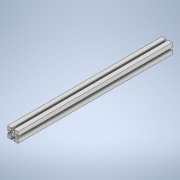
# Autodesk Inventor part: Axel_arch3
Saved by Autodesk Inventor 2020 (Build 240168000, 168)
## iProperties
Created: 2022-06-13
Part Number: Axel_arch3
Material: 일반
Document SubType Name: Modeling
Designer: samsung
Density: 1 g/cm^3
Appearance: 기본값
Author: samsung
Autodesk Inventor part; units mm, degrees
ref_plane "YZ Plane" through (0, 0, 0) normal (1, 0, 0) x (0, 1, 0)
ref_plane "XZ Plane" through (0, 0, 0) normal (0, 1, 0) x (-1, 0, 0)
ref_plane "작업 평면3" through (0, 0, 0) normal (0, 0, 1) x (1, 0, 0)
sketch "스케치4" plane through (0, 0, 0) normal (0, 0, 1) x (1, 0, 0)
  line L0 (-20, 182) -> (10, 182)
  line L1 (10, 182) -> (-20, 182)
  line L2 (-20, 182) -> (-20, 152)
  line L3 (-20, 152) -> (10, 152)
  line L4 (10, 152) -> (10, 182)
  line L5 (-20, 152) -> (-10, 152)
  line L6 (-10, 152) -> (-10, 162)
  line L7 (-10, 162) -> (-20, 162)
  line L8 (-20, 162) -> (-20, 152)
  line L9 (-20, 182) -> (-10, 182)
  line L10 (-10, 182) -> (-10, 172)
  line L11 (-10, 172) -> (-20, 172)
  line L12 (-20, 172) -> (-20, 182)
  line L13 (10, 152) -> (0, 152)
  line L14 (0, 152) -> (0, 162)
  line L15 (0, 162) -> (10, 162)
  line L16 (10, 162) -> (10, 152)
  line L17 (10, 182) -> (0, 182)
  line L18 (0, 182) -> (0, 172)
  line L19 (0, 172) -> (10, 172)
  line L20 (10, 172) -> (10, 182)
  line L21 (-18, 160) -> (-12, 160)
  line L22 (-12, 160) -> (-12, 154)
  line L23 (-12, 154) -> (-18, 154)
  line L24 (-18, 154) -> (-18, 160)
  line L25 (-18, 174) -> (-12, 174)
  line L26 (-12, 174) -> (-12, 180)
  line L27 (-12, 180) -> (-18, 180)
  line L28 (-18, 180) -> (-18, 174)
  line L29 (2, 160) -> (2, 154)
  line L30 (2, 154) -> (8, 154)
  line L31 (8, 154) -> (8, 160)
  line L32 (8, 160) -> (2, 160)
  line L33 (2, 174) -> (2, 180)
  line L34 (2, 180) -> (8, 180)
  line L35 (8, 180) -> (8, 174)
  line L36 (8, 174) -> (2, 174)
  line L37 (-10, 152) -> (-8, 152)
  line L38 (-8, 152) -> (-8, 154)
  line L39 (-8, 154) -> (-10, 154)
  line L40 (-10, 154) -> (-10, 152)
  line L41 (0, 152) -> (-2, 152)
  line L42 (-2, 152) -> (-2, 154)
  line L43 (-2, 154) -> (0, 154)
  line L44 (0, 154) -> (0, 152)
  line L45 (0, 182) -> (-2, 182)
  line L46 (-2, 182) -> (-2, 180)
  line L47 (-2, 180) -> (0, 180)
  line L48 (0, 180) -> (0, 182)
  line L49 (-10, 182) -> (-8, 182)
  line L50 (-8, 182) -> (-8, 180)
  line L51 (-8, 180) -> (-10, 180)
  line L52 (-10, 180) -> (-10, 182)
  line L53 (10, 162) -> (8, 162)
  line L54 (8, 162) -> (8, 164)
  line L55 (8, 164) -> (10, 164)
  line L56 (10, 164) -> (10, 162)
  line L57 (10, 172) -> (8, 172)
  line L58 (8, 172) -> (8, 170)
  line L59 (8, 170) -> (10, 170)
  line L60 (10, 170) -> (10, 172)
  line L61 (-20, 162) -> (-18, 162)
  line L62 (-18, 162) -> (-18, 164)
  line L63 (-18, 164) -> (-20, 164)
  line L64 (-20, 164) -> (-20, 162)
  line L65 (-20, 172) -> (-18, 172)
  line L66 (-18, 172) -> (-18, 170)
  line L67 (-18, 170) -> (-20, 170)
  line L68 (-20, 170) -> (-20, 172)
  line L69 (0, 162) -> (-10, 162)
  line L70 (-10, 162) -> (-10, 172)
  line L71 (-10, 172) -> (0, 172)
  line L72 (0, 172) -> (0, 162)
  line L73 (0, 162) -> (-10, 172) construction
  line L74 (-10, 162) -> (0, 172) construction
  line L75 (-8.5858, 162) -> (-10, 163.4142)
  line L76 (-10, 163.4142) -> (-11.4142, 162)
  line L77 (-11.4142, 162) -> (-10, 160.5858)
  line L78 (-10, 160.5858) -> (-8.5858, 162)
  line L79 (-8.5858, 162) -> (-11.4142, 162) construction
  line L80 (-10, 163.4142) -> (-10, 160.5858) construction
  line L81 (-8.5858, 172) -> (-10, 173.4142)
  line L82 (-10, 173.4142) -> (-11.4142, 172)
  line L83 (-11.4142, 172) -> (-10, 170.5858)
  line L84 (-10, 170.5858) -> (-8.5858, 172)
  line L85 (-8.5858, 172) -> (-11.4142, 172) construction
  line L86 (-10, 173.4142) -> (-10, 170.5858) construction
  line L87 (0, 170.5858) -> (1.4142, 172)
  line L88 (1.4142, 172) -> (0, 173.4142)
  line L89 (0, 173.4142) -> (-1.4142, 172)
  line L90 (-1.4142, 172) -> (0, 170.5858)
  line L91 (0, 170.5858) -> (0, 173.4142) construction
  line L92 (1.4142, 172) -> (-1.4142, 172) construction
  line L93 (0, 163.4142) -> (1.4142, 162)
  line L94 (1.4142, 162) -> (0, 160.5858)
  line L95 (0, 160.5858) -> (-1.4142, 162)
  line L96 (-1.4142, 162) -> (0, 163.4142)
  line L97 (0, 163.4142) -> (0, 160.5858) construction
  line L98 (1.4142, 162) -> (-1.4142, 162) construction
  line L99 (-2, 170) -> (-8, 170)
  line L100 (-8, 170) -> (-8, 164)
  line L101 (-8, 164) -> (-2, 164)
  line L102 (-2, 164) -> (-2, 170)
  point P0 (-5, 167)
  point P1 (0, 160.5858)
  point P2 (0, 173.4142)
  dimension "d19" = 30
  dimension "d20" = 10
  dimension "d21" = 10
  dimension "d22" = 10
  dimension "d23" = 10
  dimension "d24" = 10
  dimension "d25" = 10
  dimension "d26" = 10
  dimension "d27" = 10
  dimension "d28" = 2
  dimension "d29" = 2
  dimension "d30" = 2
  dimension "d31" = 2
  dimension "d32" = 2
  dimension "d33" = 2
  dimension "d34" = 2
  dimension "d35" = 2
  dimension "d36" = 2
  dimension "d37" = 2
  dimension "d38" = 2
  dimension "d39" = 2
  dimension "d40" = 2
  dimension "d41" = 2
  dimension "d42" = 2
  dimension "d43" = 2
  dimension "d44" = 2
  dimension "d45" = 2
  dimension "d46" = 2
  dimension "d47" = 2
  dimension "d98" = 2
  dimension "d99" = 2
  dimension "d100" = 2
  dimension "d101" = 2
  dimension "d102" = 2
  dimension "d103" = 2
  dimension "d104" = 2
  dimension "d105" = 2
  dimension "d116" = 2
  constraints: 206 end point, 48 parallel, 23 perpendicular, 15 horizontal, 10 midpoint, 15 other
  measures "d19" distance of L2.end L1.end
  measures "d20" distance of L7.end L6.end
  measures "d21" distance of L6.end L5.end
  measures "d22" distance of L10.end L11.end
  measures "d23" distance of L9.end L10.end
  measures "d24" distance of L14.end L15.end
  measures "d25" distance of L13.end L14.end
  measures "d26" distance of L19.end L18.end
  measures "d27" distance of L18.end L17.end
  measures "d28" distance between parallel lines of L7 L21
  measures "d29" distance between parallel lines of L11 L25
  measures "d30" distance between parallel lines of L14 L29
  measures "d31" distance between parallel lines of L18 L33
  measures "d32" distance of L39.end L38.end
  measures "d33" distance of L38.end L37.end
  measures "d34" distance of L42.end L43.end
  measures "d35" distance of L41.end L42.end
  measures "d36" distance of L47.end L46.end
  measures "d37" distance of L46.end L45.end
  measures "d38" distance of L50.end L51.end
  measures "d39" distance of L49.end L50.end
  measures "d40" distance of L54.end L55.end
  measures "d41" distance of L53.end L54.end
  measures "d42" distance of L59.end L58.end
  measures "d43" distance of L58.end L57.end
  measures "d44" distance of L63.end L62.end
  measures "d45" distance of L62.end L61.end
  measures "d46" distance of L66.end L67.end
  measures "d47" distance of L65.end L66.end
  measures "d98" distance of L75.start L75.end
  measures "d99" distance of L76.end L75.end
  measures "d100" distance of L81.start L81.end
  measures "d101" distance of L82.end L81.end
  measures "d102" distance of L87.start L87.end
  measures "d103" distance of L88.end L87.end
  measures "d104" distance of L93.start L93.end
  measures "d105" distance of L93.end L94.end
  measures "d116" distance between parallel lines of L71 L99
extrude "돌출7" add sketch "스케치4" against normal blind 127 contours L0 L10 L82 L11 L2 | L0 L50 L51 L10 | L11 L66 L67 L2 | L0 L18 L47 L46 | L81 L71 L10 | L10 L11 L82 | L63 L62 L7 L2 | L11 L70 L83 | L0 L4 L19 L88 L18 | L71 L84 L70 | L71 L90 L72 L96 L69 L75 L70 L84 | L7 L77 L6 L3 L2 | L89 L18 L71 | L71 L72 L90 | L75 L69 L70 | L70 L7 L76 | L4 L59 L58 L19 | L88 L19 L18 | L19 L87 L72 | L6 L39 L38 L3 | L7 L6 L77 | L69 L78 L6 | L93 L15 L72 | L72 L69 L96 | L69 L14 L95 | L4 L15 L54 L55 | L15 L94 L14 | L15 L4 L3 L14 L94 | L42 L43 L14 L3
sketch "스케치11" plane through (-20, 152, 0) normal (0, -1, 0) x (1, 0, 0)
  line L0 (18, 0) -> (30, 0) projected
  line L1 (18, 0) -> (18, -127) projected
  line L2 (30, -127) -> (18, -127) projected
  line L3 (30, 0) -> (30, -127) projected
  line L4 (0, 0) -> (12, 0) projected
  line L5 (0, 0) -> (0, -127) projected
  line L6 (12, -127) -> (0, -127) projected
  line L7 (12, 0) -> (12, -127) projected
  line L8 (0, 0) -> (12, 0) projected
  line L9 (30, 0) -> (30, -127) projected
  line L10 (0, 0) -> (30, 0)
  line L11 (30, 0) -> (30, -25)
  line L12 (30, -25) -> (0, -25)
  line L13 (0, -25) -> (0, 0)
  line L14 (30, -127) -> (0, -127)
  line L15 (0, -127) -> (0, -102)
  line L16 (0, -102) -> (30, -102)
  line L17 (30, -102) -> (30, -127)
  point P0 (20, 0)
  point P1 (15, -6.5)
  point P2 (15, -18.5)
  point P3 (15, -108.5)
  point P4 (15, -120.5)
  dimension "d117" = 25
  dimension "d118" = 25
  dimension "d119" = 6.5
  dimension "d120" = 6.5
  dimension "d121" = 6.5
  dimension "d122" = 6.5
  constraints: 16 end point, 4 parallel, 2 horizontal, 2 perpendicular, 2 point on line
  measures "d117" distance of L10.end L11.end
  measures "d118" distance of L14.end L15.end
  measures "d119" distance from line of point (15, -6.5) L10
  measures "d120" distance from line of L12 point (15, -18.5)
  measures "d121" distance from line of L16 point (15, -108.5)
  measures "d122" distance from line of L14 point (15, -120.5)
hole "구멍1" at (-5, 152, -6.5) at (-5, 152, -18.5) at (-5, 152, -108.5) at (-5, 152, -120.5) direction (0, 1, 0) diameter 6 end through all
sketch "스케치12" plane through (0, 0, 0) normal (0, 0, 1) x (1, 0, 0)
  line L0 (-1.4142, 162) -> (0, 160.5858) projected
  line L1 (0, 160.5858) -> (0, 154) projected
  line L2 (0, 154) -> (-2, 154) projected
  line L3 (-2, 154) -> (-2, 152) projected
  line L4 (-2, 152) -> (10, 152) projected
  line L5 (10, 152) -> (10, 164) projected
  line L6 (10, 164) -> (8, 164) projected
  line L7 (8, 164) -> (8, 162) projected
  line L8 (8, 162) -> (1.4142, 162) projected
  line L9 (1.4142, 162) -> (0, 163.4142) projected
  line L10 (0, 163.4142) -> (0, 170.5858) projected
  line L11 (0, 170.5858) -> (1.4142, 172) projected
  line L12 (1.4142, 172) -> (8, 172) projected
  line L13 (8, 172) -> (8, 170) projected
  line L14 (8, 170) -> (10, 170) projected
  line L15 (10, 170) -> (10, 182) projected
  line L16 (10, 182) -> (-2, 182) projected
  line L17 (-2, 182) -> (-2, 180) projected
  line L18 (-2, 180) -> (0, 180) projected
  line L19 (0, 180) -> (0, 173.4142) projected
  line L20 (0, 173.4142) -> (-1.4142, 172) projected
  line L21 (-1.4142, 172) -> (-8.5858, 172) projected
  line L22 (-8.5858, 172) -> (-10, 173.4142) projected
  line L23 (-10, 173.4142) -> (-10, 180) projected
  line L24 (-10, 180) -> (-8, 180) projected
  line L25 (-8, 180) -> (-8, 182) projected
  line L26 (-8, 182) -> (-20, 182) projected
  line L27 (-20, 182) -> (-20, 170) projected
  line L28 (-20, 170) -> (-18, 170) projected
  line L29 (-18, 170) -> (-18, 172) projected
  line L30 (-18, 172) -> (-11.4142, 172) projected
  line L31 (-11.4142, 172) -> (-10, 170.5858) projected
  line L32 (-10, 170.5858) -> (-10, 163.4142) projected
  line L33 (-10, 163.4142) -> (-11.4142, 162) projected
  line L34 (-11.4142, 162) -> (-18, 162) projected
  line L35 (-18, 162) -> (-18, 164) projected
  line L36 (-18, 164) -> (-20, 164) projected
  line L37 (-20, 164) -> (-20, 152) projected
  line L38 (-20, 152) -> (-8, 152) projected
  line L39 (-8, 152) -> (-8, 154) projected
  line L40 (-8, 154) -> (-10, 154) projected
  line L41 (-10, 154) -> (-10, 160.5858) projected
  line L42 (-10, 160.5858) -> (-8.5858, 162) projected
  line L43 (-8.5858, 162) -> (-1.4142, 162) projected
  line L44 (8, 180) -> (8, 174) projected
  line L45 (8, 174) -> (2, 174) projected
  line L46 (2, 174) -> (2, 180) projected
  line L47 (2, 180) -> (8, 180) projected
  line L48 (2, 160) -> (8, 160) projected
  line L49 (8, 160) -> (8, 154) projected
  line L50 (8, 154) -> (2, 154) projected
  line L51 (2, 154) -> (2, 160) projected
  line L52 (-2, 164) -> (-8, 164) projected
  line L53 (-8, 164) -> (-8, 170) projected
  line L54 (-8, 170) -> (-2, 170) projected
  line L55 (-2, 170) -> (-2, 164) projected
  line L56 (-18, 174) -> (-18, 180) projected
  line L57 (-18, 180) -> (-12, 180) projected
  line L58 (-12, 180) -> (-12, 174) projected
  line L59 (-12, 174) -> (-18, 174) projected
  line L60 (-12, 154) -> (-18, 154) projected
  line L61 (-18, 154) -> (-18, 160) projected
  line L62 (-18, 160) -> (-12, 160) projected
  line L63 (-12, 160) -> (-12, 154) projected
  point P0 (0, 0)
extrude "돌출8" add sketch "스케치12" along normal blind 261.5 contours L43 L42 L41 L40 L39 L38 L37 L36 L35 L34 L33 L32 L31 L30 L29 L28 L27 L26 L25 L24 L23 L22 L21 L20 L19 L18 L17 L16 L15 L14 L13 L12 L11 L10 L9 L8 L7 L6 L5 L4 L3 L2 L1 L0 | L44 L45 L46 L47 | L48 L49 L50 L51 | L52 L53 L54 L55 | L56 L57 L58 L59 | L60 L61 L62 L63
sketch "스케치13" plane through (-20, 152, -127) normal (0, -1, 0) x (1, 0, 0)
  line L0 (18, 388.5) -> (30, 388.5) projected
  line L1 (0, 388.5) -> (12, 388.5) projected
  point P0 (20, 127)
  point P1 (15, 354.5)
  point P2 (15, 334.5)
  dimension "d135" = 34
  dimension "d136" = 20
  measures "d135" distance from line of point (15, 354.5) L0
  measures "d136" distance of point (15, 334.5) point (15, 354.5)
hole "구멍2" at (-5, 152, 227.5) at (-5, 152, 207.5) direction (0, 1, 0) diameter 6 end through all
sketch "스케치14" plane through (0, 0, -127) normal (0, 0, -1) x (-1, 0, 0)
  line L0 (0, 160.5858) -> (1.4142, 162) projected
  line L1 (1.4142, 162) -> (8.5858, 162) projected
  line L2 (8.5858, 162) -> (10, 160.5858) projected
  line L3 (10, 160.5858) -> (10, 154) projected
  line L4 (10, 154) -> (8, 154) projected
  line L5 (8, 154) -> (8, 152) projected
  line L6 (8, 152) -> (20, 152) projected
  line L7 (20, 152) -> (20, 164) projected
  line L8 (20, 164) -> (18, 164) projected
  line L9 (18, 164) -> (18, 162) projected
  line L10 (18, 162) -> (11.4142, 162) projected
  line L11 (11.4142, 162) -> (10, 163.4142) projected
  line L12 (10, 163.4142) -> (10, 170.5858) projected
  line L13 (10, 170.5858) -> (11.4142, 172) projected
  line L14 (11.4142, 172) -> (18, 172) projected
  line L15 (18, 172) -> (18, 170) projected
  line L16 (18, 170) -> (20, 170) projected
  line L17 (20, 170) -> (20, 182) projected
  line L18 (20, 182) -> (8, 182) projected
  line L19 (8, 182) -> (8, 180) projected
  line L20 (8, 180) -> (10, 180) projected
  line L21 (10, 180) -> (10, 173.4142) projected
  line L22 (10, 173.4142) -> (8.5858, 172) projected
  line L23 (8.5858, 172) -> (1.4142, 172) projected
  line L24 (1.4142, 172) -> (0, 173.4142) projected
  line L25 (0, 173.4142) -> (0, 180) projected
  line L26 (0, 180) -> (2, 180) projected
  line L27 (2, 180) -> (2, 182) projected
  line L28 (2, 182) -> (-10, 182) projected
  line L29 (-10, 182) -> (-10, 170) projected
  line L30 (-10, 170) -> (-8, 170) projected
  line L31 (-8, 170) -> (-8, 172) projected
  line L32 (-8, 172) -> (-1.4142, 172) projected
  line L33 (-1.4142, 172) -> (0, 170.5858) projected
  line L34 (0, 170.5858) -> (0, 163.4142) projected
  line L35 (0, 163.4142) -> (-1.4142, 162) projected
  line L36 (-1.4142, 162) -> (-8, 162) projected
  line L37 (-8, 162) -> (-8, 164) projected
  line L38 (-8, 164) -> (-10, 164) projected
  line L39 (-10, 164) -> (-10, 152) projected
  line L40 (-10, 152) -> (2, 152) projected
  line L41 (2, 152) -> (2, 154) projected
  line L42 (2, 154) -> (0, 154) projected
  line L43 (0, 154) -> (0, 160.5858) projected
  line L44 (-8, 174) -> (-8, 180) projected
  line L45 (-8, 180) -> (-2, 180) projected
  line L46 (-2, 180) -> (-2, 174) projected
  line L47 (-2, 174) -> (-8, 174) projected
  line L48 (-8, 160) -> (-2, 160) projected
  line L49 (-2, 160) -> (-2, 154) projected
  line L50 (-2, 154) -> (-8, 154) projected
  line L51 (-8, 154) -> (-8, 160) projected
  line L52 (8, 164) -> (2, 164) projected
  line L53 (2, 164) -> (2, 170) projected
  line L54 (2, 170) -> (8, 170) projected
  line L55 (8, 170) -> (8, 164) projected
  line L56 (18, 180) -> (18, 174) projected
  line L57 (18, 174) -> (12, 174) projected
  line L58 (12, 174) -> (12, 180) projected
  line L59 (12, 180) -> (18, 180) projected
  line L60 (18, 154) -> (12, 154) projected
  line L61 (12, 154) -> (12, 160) projected
  line L62 (12, 160) -> (18, 160) projected
  line L63 (18, 160) -> (18, 154) projected
  point P0 (0, 0)
extrude "돌출9" add sketch "스케치14" along normal blind 61.5
